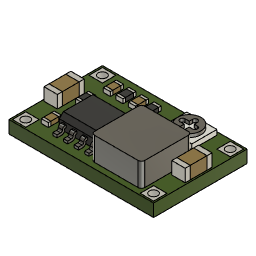
Mini360 DC-DC buck v2 (Autodesk Fusion 360 design; units mm, degrees)
Autodesk Fusion 360 part; units mm, degrees
sketch "Sketch1" plane through (0, 0, 0) normal (0, 0, 1) x (1, 0, 0) in component "Mini360 Voltage Buck"
  circle A0 centre (-7.62, 4.572) radius 0.5
  circle A1 centre (7.62, 4.572) radius 0.5
  circle A2 centre (-7.62, -4.572) radius 0.5
  circle A3 centre (7.62, -4.572) radius 0.5
  line L0 (-8.62, 5.572) -> (8.62, 5.572)
  line L1 (8.62, 5.572) -> (8.62, -5.572)
  line L2 (8.62, -5.572) -> (-8.62, -5.572)
  line L3 (-8.62, -5.572) -> (-8.62, 5.572)
  line L4 (-4.7, 0.5) -> (0.3, 0.5)
  line L5 (0.3, 0.5) -> (0.3, -3.5)
  line L6 (0.3, -3.5) -> (-4.7, -3.5)
  line L7 (-4.7, -3.5) -> (-4.7, 0.5)
  line L8 (-4.35, -3.5) -> (-3.85, -3.5)
  line L9 (-3.85, -3.5) -> (-3.85, -4.6)
  line L10 (-3.85, -4.6) -> (-4.35, -4.6)
  line L11 (-4.35, -4.6) -> (-4.35, -3.5)
  line L12 (-3.08, -4.6) -> (-3.08, -3.5)
  line L13 (-3.08, -3.5) -> (-2.58, -3.5)
  line L14 (-2.58, -3.5) -> (-2.58, -4.6)
  line L15 (-2.58, -4.6) -> (-3.08, -4.6)
  line L16 (-1.81, -4.6) -> (-1.81, -3.5)
  line L17 (-1.81, -3.5) -> (-1.31, -3.5)
  line L18 (-1.31, -3.5) -> (-1.31, -4.6)
  line L19 (-1.31, -4.6) -> (-1.81, -4.6)
  line L20 (-0.54, -4.6) -> (-0.54, -3.5)
  line L21 (-0.54, -3.5) -> (-0.04, -3.5)
  line L22 (-0.04, -3.5) -> (-0.04, -4.6)
  line L23 (-0.04, -4.6) -> (-0.54, -4.6)
  line L24 (-4.35, -4.6) -> (-4.35, -3.5)
  line L25 (-4.35, -3.5) -> (-3.85, -3.5)
  line L26 (-3.85, -3.5) -> (-3.85, -4.6)
  line L27 (-3.85, -4.6) -> (-4.35, -4.6)
  line L28 (-3.85, 0.5) -> (-4.35, 0.5)
  line L29 (-2.58, 1.6) -> (-2.58, 0.5)
  line L30 (-1.81, 0.5) -> (-1.81, 1.6)
  line L31 (-2.58, 0.5) -> (-3.08, 0.5)
  line L32 (-0.54, 1.6) -> (-0.04, 1.6)
  line L33 (-3.08, 1.6) -> (-2.58, 1.6)
  line L34 (-1.31, 1.6) -> (-1.31, 0.5)
  line L35 (-3.85, 1.6) -> (-3.85, 0.5)
  line L36 (-4.35, 0.5) -> (-4.35, 1.6)
  line L37 (-0.04, 0.5) -> (-0.54, 0.5)
  line L38 (-1.81, 1.6) -> (-1.31, 1.6)
  line L39 (-1.31, 0.5) -> (-1.81, 0.5)
  line L40 (-0.54, 0.5) -> (-0.54, 1.6)
  line L41 (-3.85, 0.5) -> (-4.35, 0.5)
  line L42 (-0.04, 1.6) -> (-0.04, 0.5)
  line L43 (-3.85, 1.6) -> (-3.85, 0.5)
  line L44 (-3.08, 0.5) -> (-3.08, 1.6)
  line L45 (-4.35, 1.6) -> (-3.85, 1.6)
  line L46 (-4.35, 1.6) -> (-3.85, 1.6)
  line L47 (-4.35, 0.5) -> (-4.35, 1.6)
  line L48 (0.5, 1.1) -> (6.5, 1.1)
  line L49 (6.5, 1.1) -> (6.5, -4.9)
  line L50 (6.5, -4.9) -> (0.5, -4.9)
  line L51 (0.5, -4.9) -> (0.5, 1.1)
  line L52 (6.82, 1.6) -> (8.42, 1.6)
  line L53 (8.42, 1.6) -> (8.42, -1.6)
  line L54 (8.42, -1.6) -> (6.82, -1.6)
  line L55 (6.82, -1.6) -> (6.82, 1.6)
  line L56 (-6.82, -3.772) -> (-6.82, -5.372)
  line L57 (-6.82, -5.372) -> (-8.42, -5.372)
  line L58 (-8.42, -5.372) -> (-8.42, -3.772)
  line L59 (-8.42, -3.772) -> (-6.82, -3.772)
  line L60 (-8.42, 3.772) -> (-8.42, 5.372)
  line L61 (-8.42, 5.372) -> (-6.82, 5.372)
  line L62 (-6.82, 5.372) -> (-6.82, 3.772)
  line L63 (-6.82, 3.772) -> (-8.42, 3.772)
  line L64 (6.82, 3.772) -> (6.82, 5.372)
  line L65 (6.82, 5.372) -> (8.42, 5.372)
  line L66 (8.42, 5.372) -> (8.42, 3.772)
  line L67 (8.42, 3.772) -> (6.82, 3.772)
  line L68 (6.82, -5.372) -> (6.82, -3.772)
  line L69 (6.82, -3.772) -> (8.42, -3.772)
  line L70 (8.42, -5.372) -> (6.82, -5.372)
  line L71 (8.42, -3.772) -> (8.42, -5.372)
  line L72 (-6.82, 1.6) -> (-6.82, -1.6)
  line L73 (-6.82, -1.6) -> (-8.42, -1.6)
  line L74 (-8.42, -1.6) -> (-8.42, 1.6)
  line L75 (-8.42, 1.6) -> (-6.82, 1.6)
  line L76 (-5.8, 4.4) -> (-4.95, 4.4)
  line L77 (-4.95, 4.4) -> (-4.95, 2.85)
  line L78 (-4.95, 2.85) -> (-5.8, 2.85)
  line L79 (-5.8, 2.85) -> (-5.8, 4.4)
  line L80 (-5.8, 2.85) -> (-5.8, 4.4)
  line L81 (-5.8, 4.4) -> (-4.95, 4.4)
  line L82 (-4.95, 4.4) -> (-4.95, 2.85)
  line L83 (-4.95, 2.85) -> (-5.8, 2.85)
  line L84 (-3.45, 4.4) -> (-3.45, 2.85)
  line L85 (-3.45, 2.85) -> (-4.3, 2.85)
  line L86 (-4.3, 2.85) -> (-4.3, 4.4)
  line L87 (-4.3, 4.4) -> (-3.45, 4.4)
  line L88 (-1.95, 4.4) -> (-1.95, 2.85)
  line L89 (-1.95, 2.85) -> (-2.8, 2.85)
  line L90 (-2.8, 2.85) -> (-2.8, 4.4)
  line L91 (-2.8, 4.4) -> (-1.95, 4.4)
  line L92 (-0.45, 4.4) -> (-0.45, 2.85)
  line L93 (-0.45, 2.85) -> (-1.3, 2.85)
  line L94 (-1.3, 2.85) -> (-1.3, 4.4)
  line L95 (-1.3, 4.4) -> (-0.45, 4.4)
  circle A4 centre (3.6, 3.7) radius 1.4
  line L96 (1.8, 5.2) -> (5.4, 5.2)
  line L97 (5.4, 5.2) -> (5.4, 2.2)
  line L98 (5.4, 2.2) -> (1.8, 2.2)
  line L99 (1.8, 2.2) -> (1.8, 5.2)
  arc A5 (3.3, 2.9) -> (3.9, 2.9) centre (3.6, 2.9) ccw
  arc A6 (3.9, 4.4) -> (3.3, 4.4) centre (3.6, 4.4) ccw
  arc A7 (2.8, 4) -> (2.8, 3.4) centre (2.8, 3.7) ccw
  arc A8 (4.3, 3.4) -> (4.3, 4) centre (4.3, 3.7) ccw
  line L100 (4.3, 4) -> (3.9, 4)
  line L101 (3.3, 4) -> (2.8, 4)
  line L102 (3.9, 4) -> (3.9, 4.4)
  line L103 (2.8, 3.4) -> (3.3, 3.4)
  line L104 (3.9, 3.4) -> (4.3, 3.4)
  line L105 (3.3, 4.4) -> (3.3, 4)
  line L106 (3.3, 3.4) -> (3.3, 2.9)
  line L107 (3.9, 3.4) -> (3.9, 2.9)
  line L108 (-6.3, 0.05) -> (-6.3, 1.6)
  line L109 (-6.3, 1.6) -> (-5.45, 1.6)
  line L110 (-5.45, 1.6) -> (-5.45, 0.05)
  line L111 (-5.45, 0.05) -> (-6.3, 0.05)
  line L112 (-6.3, -4.05) -> (-6.3, -2.5)
  line L113 (-6.3, -2.5) -> (-5.45, -2.5)
  line L114 (-5.45, -2.5) -> (-5.45, -4.05)
  line L115 (-5.45, -4.05) -> (-6.3, -4.05)
  line L116 (8.42, 1) -> (6.82, 1)
  line L117 (8.42, -1) -> (6.82, -1)
  line L118 (-6.82, 1) -> (-8.42, 1)
  line L119 (-6.82, -1) -> (-8.42, -1)
  line L120 (-5.8, 4.1) -> (-4.95, 4.1)
  line L121 (-4.3, 4.1) -> (-3.45, 4.1)
  line L122 (-5.8, 3.15) -> (-4.95, 3.15)
  line L123 (-4.3, 3.15) -> (-3.45, 3.15)
  line L124 (-2.8, 3.15) -> (-1.95, 3.15)
  line L125 (-1.3, 3.15) -> (-0.45, 3.15)
  line L126 (-2.8, 4.1) -> (-1.95, 4.1)
  line L127 (-1.3, 4.1) -> (-0.45, 4.1)
  line L128 (-6.3, 0.35) -> (-5.45, 0.35)
  line L129 (-6.3, 1.3) -> (-5.45, 1.3)
  line L130 (-6.3, -3.75) -> (-5.45, -3.75)
  line L131 (-6.3, -2.8) -> (-5.45, -2.8)
  line L132 (-4.35, 0.7) -> (-3.85, 0.7)
  line L133 (-4.35, 0.95) -> (-3.85, 0.95)
  dimension "d30" = 6
  dimension "d31" = 6
  dimension "d32" = 1.6
  dimension "d33" = 3.2
  dimension "d34" = 17.24
  dimension "d35" = 11.144
  dimension "d41" = 15.24
  dimension "d43" = 9.144
  dimension "d44" = 1.6
  dimension "d45" = 3.2
  dimension "d51" = 3.6
  dimension "d52" = 3
  constraint horizontal L4
  constraint vertical L5
  constraint horizontal L6
  constraint vertical L7
  constraint horizontal L8
  constraint vertical L9
  constraint horizontal L10
  constraint vertical L11
  constraint horizontal L13
  constraint vertical L14
  constraint horizontal L15
  constraint vertical L12
  constraint horizontal L17
  constraint vertical L18
  constraint horizontal L19
  constraint vertical L16
  constraint horizontal L21
  constraint vertical L22
  constraint horizontal L23
  constraint vertical L20
  constraint horizontal L25
  constraint vertical L26
  constraint horizontal L27
  constraint vertical L24
  constraint horizontal L45
  constraint vertical L35
  constraint horizontal L28
  constraint vertical L36
  constraint horizontal L33
  constraint vertical L29
  constraint horizontal L31
  constraint vertical L44
  constraint horizontal L38
  constraint vertical L34
  constraint horizontal L39
  constraint vertical L30
  constraint horizontal L32
  constraint vertical L42
  constraint horizontal L37
  constraint vertical L40
  constraint horizontal L46
  constraint vertical L43
  constraint horizontal L41
  constraint vertical L47
  constraint horizontal L48
  constraint vertical L49
  constraint horizontal L50
  constraint vertical L51
  constraint horizontal L52
  constraint vertical L53
  constraint horizontal L54
  constraint vertical L55
  constraint horizontal L75
  constraint vertical L72
  constraint horizontal L73
  constraint vertical L74
  constraint horizontal L76
  constraint vertical L77
  constraint horizontal L78
  constraint vertical L79
  constraint horizontal L81
  constraint vertical L82
  constraint horizontal L83
  constraint vertical L80
  constraint horizontal L87
  constraint vertical L84
  constraint horizontal L85
  constraint vertical L86
  constraint horizontal L91
  constraint vertical L88
  constraint horizontal L89
  constraint vertical L90
  constraint horizontal L95
  constraint vertical L92
  constraint horizontal L93
  constraint vertical L94
  constraint horizontal L96
  constraint vertical L97
  constraint horizontal L98
  constraint vertical L99
  constraint tangent A7 L103
  constraint coincident L103.end L105
  constraint tangent A5 L107
  constraint horizontal L109
  constraint vertical L110
  constraint horizontal L111
  constraint vertical L108
  constraint horizontal L113
  constraint vertical L114
  constraint horizontal L115
  constraint vertical L112
  constraint coincident L55 L116.end
  constraint perpendicular L55 L116
  constraint coincident L55 L117.end
  constraint perpendicular L55 L117
  constraint coincident L53 L116.start
  constraint coincident L53 L117.start
  constraint coincident L74 L118.end
  constraint perpendicular L74 L118
  constraint coincident L74 L119.end
  constraint perpendicular L74 L119
  constraint coincident L72 L119.start
  constraint coincident L72 L118.start
  constraint coincident L92 L127.end
  constraint coincident L92 L125.end
  constraint coincident L86 L123.start
  constraint coincident L88 L124.end
  constraint coincident L94 L125.start
  constraint coincident L94 L127.start
  constraint coincident L43 L132.end
  constraint perpendicular L43 L132
  constraint coincident L35 L133.end
  constraint perpendicular L35 L133
  constraint coincident L36 L132.start
  constraint coincident L36 L133.start
  measures "d30" distance of L48.start L48.end
  measures "d31" distance of L48.start L50.end
  measures "d32" distance of L52.start L52.end
  measures "d33" distance of L52.start L54.end
  measures "d34" distance of L0.start L0.end
  measures "d35" distance of L0.start L2.end
  measures "d41" distance of A0.centre A1.centre
  measures "d43" distance of A0.centre A2.centre
  measures "d44" distance of L72.start L74.end
  measures "d45" distance of L73.end L74.end
  measures "d51" distance of L96.start L96.end
  measures "d52" distance of L96.start L98.end
extrude "Extrude1" add sketch "Sketch1" along normal blind 1.5 contours A0 | A1 | A2 | A3 | L0 L1 L2 L3 | L4 L5 L6 L7 L8 L13 L17 L21 L25 L28 L31 L37 L39 L41 | L4 L28 L35 L36 L41 L43 L47 L132 | L35 L36 L43 L47 L132 L133 | L6 L8 L9 L10 L11 L24 L25 L26 L27 | L4 L29 L31 L33 L44 | L35 L36 L43 L45 L46 L47 L133 | L6 L12 L13 L14 L15 | L4 L30 L34 L38 L39 | L6 L16 L17 L18 L19 | L4 L32 L37 L40 L42 | L6 L20 L21 L22 L23 | L48 L49 L50 L51 | L52 L53 L55 L116 | L53 L55 L116 L117 | L53 L54 L55 L117 | L56 L57 L58 L59 | L60 L61 L62 L63 | L64 L65 L66 L67 | L68 L69 L70 L71 | L72 L74 L75 L118 | L72 L74 L118 L119 | L72 L73 L74 L119 | L76 L77 L79 L80 L81 L82 L120 | L77 L79 L80 L82 L120 L122 | L77 L78 L79 L80 L82 L83 L122 | L84 L86 L87 L121 | L84 L86 L121 L123 | L84 L85 L86 L123 | L88 L90 L91 L126 | L88 L90 L124 L126 | L88 L89 L90 L124 | L92 L94 L95 L127 | L92 L94 L125 L127 | L92 L93 L94 L125 | A4 | L96 L97 L98 L99 | A5 A6 A7 A8 L100 L101 L102 L103 L104 L105 L106 L107 | L108 L110 L111 L128 | L108 L110 L128 L129 | L108 L109 L110 L129 | L112 L114 L115 L130 | L112 L114 L130 L131 | L112 L113 L114 L131 makes body 1 in component "Mini360 Voltage Buck"
extrude "Extrude2" cut sketch "Sketch1" along normal blind 2 contours A0 | A1 | A2 | A3 | L56 L57 L58 L59 | L60 L61 L62 L63 | L64 L65 L66 L67 | L68 L69 L70 L71 bodies 1 in component "Mini360 Voltage Buck"
extrude "Extrude3" add sketch "Sketch1" along normal blind 1.5 separate body contours L56 L57 L58 L59 | L60 L61 L62 L63 | L64 L65 L66 L67 | L68 L69 L70 L71 makes body 2 at (-7.1206, 4.5471, 1) makes body 3 at (8.1194, 4.5471, 1) makes body 4 at (-7.1206, -4.5969, 1) makes body 5 at (8.1194, -4.5969, 1) in component "Mini360 Voltage Buck"
extrude "Extrude4" add sketch "Sketch1" along normal blind 3 and the other way blind -1.5 separate body contours L53 L55 L116 L117 | L72 L74 L118 L119 makes body 6 at (7.3533, -0.3333, 1.5) makes body 7 at (-7.8867, 0.3333, 1.5) in component "Mini360 Voltage Buck"
extrude "Extrude5" add sketch "Sketch1" along normal blind 3 and the other way blind -1.5 separate body contours L52 L53 L55 L116 | L53 L54 L55 L117 | L72 L74 L75 L118 | L72 L73 L74 L119 makes body 8 at (7.8867, 1, 2) makes body 9 at (-7.3533, -1.6, 2) makes body 10 at (7.8867, -1, 2) makes body 11 at (-7.3533, 1, 2) in component "Mini360 Voltage Buck"
extrude "Extrude6" add sketch "Sketch1" along normal blind 4.3 and the other way blind -1.5 separate body contours L48 L49 L50 L51 makes body 12 in component "Mini360 Voltage Buck"
extrude "Extrude7" add sketch "Sketch1" along normal blind 3 and the other way blind -1.5 separate body contours L4 L5 L6 L7 L8 L13 L17 L21 L25 L28 L31 L37 L39 L41 makes body 13 in component "Mini360 Voltage Buck"
extrude "Extrude8" add sketch "Sketch1" along normal blind 2 and the other way blind -1.5 separate body contours L77 L79 L80 L82 L120 L122 | L84 L86 L121 L123 | L88 L90 L124 L126 | L92 L94 L125 L127 | L108 L110 L128 L129 | L112 L114 L130 L131 makes body 14 at (-4.0167, 3.7833, 1.5) makes body 15 at (-6.0167, -3.1167, 1.5) makes body 16 at (-2.5167, 3.7833, 1.5) makes body 17 at (-5.5167, 3.7833, 1.5) makes body 18 at (-6.0167, 0.9833, 1.5) makes body 19 at (-1.0167, 3.7833, 1.5) in component "Mini360 Voltage Buck"
extrude "Extrude9" add sketch "Sketch1" along normal blind 2 and the other way blind -1.5 separate body contours L76 L77 L79 L80 L81 L82 L120 | L77 L78 L79 L80 L82 L83 L122 | L84 L86 L87 L121 | L84 L85 L86 L123 | L88 L90 L91 L126 | L88 L89 L90 L124 | L92 L94 L95 L127 | L92 L93 L94 L125 | L108 L110 L111 L128 | L108 L109 L110 L129 | L112 L114 L115 L130 | L112 L113 L114 L131 makes body 20 at (-2.5167, 4.1, 1.6667) makes body 21 at (-5.5167, 4.4, 1.6667) makes body 22 at (-6.0167, -2.5, 1.6667) makes body 23 at (-6.0167, 0.35, 1.6667) makes body 24 at (-4.0167, 4.1, 1.6667) makes body 25 at (-0.7333, 4.4, 1.8333) makes body 26 at (-2.2333, 2.85, 1.6667) makes body 27 at (-5.5167, 3.15, 1.6667) makes body 28 at (-6.0167, -3.75, 1.6667) makes body 29 at (-6.0167, 1.6, 1.6667) makes body 30 at (-3.7333, 2.85, 1.6667) makes body 31 at (-1.0167, 2.85, 1.8333) in component "Mini360 Voltage Buck"
extrude "Extrude10" add sketch "Sketch1" along normal blind 2.3 and the other way blind -2 separate body contours L4 L28 L35 L36 L41 L43 L47 L132 makes body 32 in component "Mini360 Voltage Buck"
extrude "Extrude11" add sketch "Sketch1" along normal blind 2.3 and the other way blind -1.5 contours L35 L36 L43 L47 L132 L133 bodies 32 in component "Mini360 Voltage Buck"
extrude "Extrude12" add sketch "Sketch1" along normal blind 1.8 and the other way blind -1.5 contours L35 L36 L43 L45 L46 L47 L133 bodies 32 in component "Mini360 Voltage Buck"
fillet "Fillet1" radius 0.3 1 edges at (-4.1, 0.95, 2.3) on bodies 32 in component "Mini360 Voltage Buck"
fillet "Fillet2" radius 0.075 1 edges at (-4.1, 0.7, 2) on bodies 32 in component "Mini360 Voltage Buck"
fillet "Fillet3" radius 0.35 1 edges at (-4.1, 0.7, 1.5) on bodies 32 in component "Mini360 Voltage Buck"
fillet "Fillet4" radius 0.2 1 edges at (-4.1, 0.95, 1.8) on bodies 32 in component "Mini360 Voltage Buck"
copy_body "CopyPasteBodies1" bodies 32 makes body 33 in component "Mini360 Voltage Buck"
move_body "Move1" bodies 33 to x (1, 0, 0) y (0, 1, 0) z (0, 0, 1) at (1.27, 0, 0) in component "Mini360 Voltage Buck"
copy_body "CopyPasteBodies2" bodies 32 makes body 34 in component "Mini360 Voltage Buck"
move_body "Move2" bodies 34 to x (1, 0, 0) y (0, 1, 0) z (0, 0, 1) at (2.54, 0, 0) in component "Mini360 Voltage Buck"
copy_body "CopyPasteBodies3" bodies 32 makes body 35 in component "Mini360 Voltage Buck"
move_body "Move3" bodies 35 to x (1, 0, 0) y (0, 1, 0) z (0, 0, 1) at (3.81, 0, 0) in component "Mini360 Voltage Buck"
copy_body "CopyPasteBodies4" bodies 32 33 34 35 makes body 36 makes body 37 makes body 38 makes body 39 in component "Mini360 Voltage Buck"
move_body "Move4" bodies 36 37 38 39 to x (-1, 0, 0) y (0, -1, 0) z (0, 0, 1) at (-4.4, -3, 0) in component "Mini360 Voltage Buck"
fillet "Fillet5" radius 0.4 4 edges at (6.5, -4.9, 2.9) (0.5, -4.9, 2.9) (0.5, 1.1, 2.9) (6.5, 1.1, 2.9) on bodies 12 in component "Mini360 Voltage Buck"
chamfer "Chamfer1" distance 0.5 angle 45 1 edges at (-2.2, -3.5, 3) on bodies 13 in component "Mini360 Voltage Buck"
extrude "Extrude13" add sketch "Sketch1" along normal blind 2.1 and the other way blind -1.5 separate body contours A4 | L96 L97 L98 L99 | A5 A6 A7 A8 L100 L101 L102 L103 L104 L105 L106 L107 makes body 40 in component "Mini360 Voltage Buck"
extrude "Extrude14" add sketch "Sketch1" along normal blind 2.5 and the other way blind -2.1 separate body contours A4 makes body 41 in component "Mini360 Voltage Buck"
component "Mini360 Voltage Buck" placed x (1, 0, 0) y (0, 1, 0) z (0, 0, 1) at (0, 0, 0)
